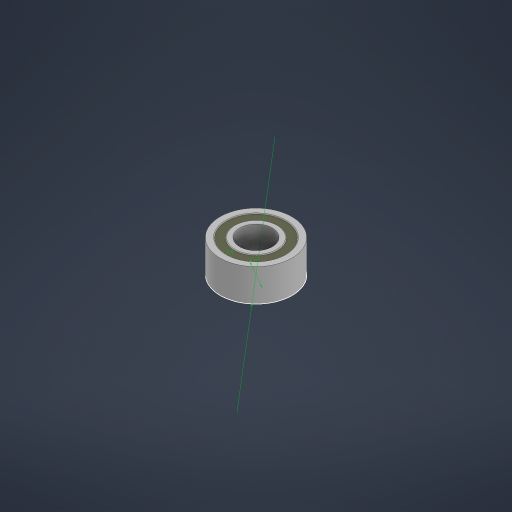
# Autodesk Inventor part: Bearing 5mmID
Saved by Autodesk Inventor 2024 (Build 280153000, 153)
## iProperties
Created: 2024-10-26
Part Number: Bearing 5mmID
Material: Generic
Document SubType Name: Modeling
Designer: jerem
Density: 1 g/cm^3
Appearance: Default
Author: jerem
Autodesk Inventor part; units mm, degrees
ref_plane "YZ Plane" through (0, 0, 0) normal (1, 0, 0) x (0, 1, 0)
ref_plane "XZ Plane" through (0, 0, 0) normal (0, 1, 0) x (-1, 0, 0)
ref_plane "XY Plane" through (0, 0, 0) normal (0, 0, 1) x (1, 0, 0)
sketch "Sketch1" plane through (0, 0, 0) normal (0, 1, 0) x (-1, 0, 0)
  circle A0 centre (0, 0) radius 5.5
  circle A1 centre (0, 0) radius 2.5
  circle A2 centre (0, 0) radius 3.2
  circle A3 centre (0, 0) radius 4.6
  dimension "d0" = 11
  dimension "d1" = 5
  dimension "d2" = 0.9
  dimension "d3" = 0.7
  constraints: 4 centre point, 4 coincident
  measures "d0" diameter of A0
  measures "d1" diameter of A1
  measures "d2" radial gap between concentric circles of A0 A3
  measures "d3" radial gap between concentric circles of A1 A2
extrude "Extrusion1" add sketch "Sketch1" along normal blind 4.95 contours A0 | A2 | A3
extrude "Extrusion2" cut sketch "Sketch1" along normal blind 0.1 contours A3
extrude "Extrusion3" cut sketch "Sketch1" against normal blind 0.1 from surface at 4.95 contours A3
fillet "Fillet1" radius 0.1 4 edges at (4.6, 0.1, 0) (3.2, 0.1, 0) (3.2, 4.85, 0) (4.6, 4.85, 0) inverted yes
body "Solid1"
